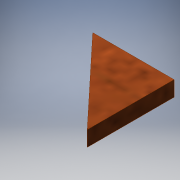
# Autodesk Inventor part: acople 4
Saved by Autodesk Inventor 2016 (Build 200138000, 138)
## iProperties
Created: 2016-08-02
Part Number: acople 4
Material: Madera (nogal)
Document SubType Name: Modeling
Designer: DanielFelipe
Density: 0.55 g/cm^3
Appearance: Nogal - Natural pulido
Mass: 0.22321 g
Surface Area: 4.39165 cm^2
Volume: 0.405837 cm^3
Author: DanielFelipe
Autodesk Inventor part; units mm, degrees
ref_plane "YZ Plane" through (0, 0, 0) normal (1, 0, 0) x (0, 1, 0)
ref_plane "XZ Plane" through (0, 0, 0) normal (0, 1, 0) x (-1, 0, 0)
ref_plane "XY Plane" through (0, 0, 0) normal (0, 0, 1) x (1, 0, 0)
sketch "Boceto1" plane through (0, 0, 0) normal (0, 0, 1) x (1, 0, 0)
  line L0 (-15.9152, 17) -> (0, 17)
  line L1 (0, 0) -> (0, 17)
  line L2 (0, 0) -> (-15.9152, 17)
  point P0 (0, 0)
  constraints: 6 end point
extrude "Extrusión1" add sketch "Boceto1" along normal blind 3
